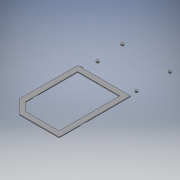
# Autodesk Inventor part: Backplate_V2
Saved by Autodesk Inventor 2016 SP2 (Build 200236200, 236)
## iProperties
Created: 2018-06-11
Part Number: Backplate_V2
Material: Generisch
Document SubType Name: Modeling
Designer: Nils
Density: 1 g/cm^3
Appearance: Vorgabe
Author: Nils
Autodesk Inventor part; units mm, degrees
ref_plane "YZ Plane" through (0, 0, 0) normal (1, 0, 0) x (0, 1, 0)
ref_plane "XZ Plane" through (0, 0, 0) normal (0, 1, 0) x (-1, 0, 0)
ref_plane "XY Plane" through (0, 0, 0) normal (0, 0, 1) x (1, 0, 0)
sketch "Skizze1" plane through (0, 0, 0) normal (0, 0, 1) x (1, 0, 0)
  line L0 (49.5001, 248.3761) -> (-49.5001, 248.3761) projected
  line L1 (49.5001, 95.1751) -> (49.5001, 248.3761) projected
  line L2 (-49.5001, 248.3761) -> (-49.5001, 95.1751) construction
  line L3 (-49.5001, 95.1751) -> (49.5001, 95.1751) construction
  line L4 (49.5001, 95.1751) -> (-20.5915, 95.1751)
  line L5 (-20.5915, 95.1751) -> (-49.5001, 124.0836)
  line L6 (-49.5001, 124.0836) -> (-49.5001, 248.3761)
  line L7 (-39.5001, 238.3761) -> (39.5001, 238.3761)
  line L8 (39.5001, 238.3761) -> (39.5001, 105.1751)
  line L9 (39.5001, 105.1751) -> (-19.2778, 105.1751)
  line L10 (-19.2778, 105.1751) -> (-39.5001, 125.3973)
  line L11 (-39.5001, 125.3973) -> (-39.5001, 238.3761)
  circle A0 centre (44.5001, 243.3761) radius 2.5 projected
  circle A1 centre (-44.5001, 243.3761) radius 2.5 projected
  circle A2 centre (-44.5001, 171.4345) radius 2.5 projected
  circle A3 centre (44.5001, 171.4345) radius 2.5 projected
  circle A4 centre (44.5001, 100.1751) radius 2.5 projected
  circle A5 centre (-20.9666, 110.5265) radius 1.75 projected
  circle A6 centre (-24.6237, 114.0565) radius 1.75 projected
  circle A7 centre (-44.8001, 100.0237) radius 1.75 projected
  circle A8 centre (-29.7001, 100.0237) radius 1.75 projected
  point P0 (0, 0)
  dimension "d0" = 135
  dimension "d1" = 8
  dimension "d3" = 10
  dimension "d4" = 10
  dimension "d5" = 10
  dimension "d6" = 10
  dimension "d22" = 2.5
  constraints: 16 end point, 3 perpendicular, 2 point on line, 1 collinear, 1 horizontal, 1 parallel
  measures "d0" angle of L5 L3
  measures "d1" distance between parallel lines of L5 L10
  measures "d3" distance between parallel lines of L3 L9
  measures "d4" distance between parallel lines of L1 L8
  measures "d5" distance between parallel lines of L2 L11
  measures "d6" distance between parallel lines of L0 L7
  measures "d22" distance from line of A6.centre L10
extrude "Extrusion1" add sketch "Skizze1" along normal blind 1.5 contours L1 L4 L5 L6 L0 | A0 | A1 | A2 | A3 | A4
sketch "Skizze2" plane through (0, 0, 0) normal (0, 0, -1) x (-1, 0, 0)
  circle A0 centre (-44.5001, 100.1751) radius 2.5 projected
  circle A1 centre (-44.5001, 171.4345) radius 2.5 projected
  circle A2 centre (-44.5001, 243.3761) radius 2.5 projected
  circle A3 centre (40.1569, 120.3973) radius 2.5 projected
  circle A4 centre (44.5001, 171.4345) radius 2.5 projected
  circle A5 centre (44.5001, 243.3761) radius 2.5 projected
  circle A6 centre (-44.5001, 100.1751) radius 2.4
  circle A7 centre (-44.5001, 171.4345) radius 2.4
  circle A8 centre (-44.5001, 243.3761) radius 2.4
  circle A9 centre (44.5001, 243.3761) radius 2.4
  circle A10 centre (44.5001, 171.4345) radius 2.4
  circle A11 centre (40.1569, 120.3973) radius 2.4
  dimension "d23" = 0.1
  dimension "d24" = 4.8
  dimension "d25" = 4.8
  dimension "d26" = 4.8
  dimension "d27" = 4.8
  dimension "d28" = 4.8
  dimension "d29" = 4.8
  constraints: 6 centre point, 5 coincident
  measures "d23" radial gap between concentric circles of A0 A6
  measures "d24" diameter of A6
  measures "d25" diameter of A7
  measures "d26" diameter of A8
  measures "d27" diameter of A9
  measures "d28" diameter of A10
  measures "d29" diameter of A11
extrude "Extrusion2" add sketch "Skizze2" along normal blind 2.6 contours A6 | A7 | A8 | A9 | A10 | A11
sketch "Skizze3" plane through (0, 0, 0) normal (0, 0, -1) x (-1, 0, 0)
  line L0 (-49.5001, 95.1751) -> (-49.5001, 248.3761) projected
  line L1 (-39.5001, 238.3761) -> (-39.5001, 105.1751) projected
  line L2 (-49.5001, 135.1751) -> (-39.5001, 135.1751)
  line L3 (-39.5001, 135.1751) -> (-39.5001, 145.1751)
  line L4 (-39.5001, 145.1751) -> (-49.5001, 145.1751)
  line L5 (-49.5001, 145.1751) -> (-49.5001, 135.1751)
  line L6 (39.5001, 238.3761) -> (39.5001, 125.3973) projected
  line L7 (49.5001, 248.3761) -> (49.5001, 124.0836) projected
  line L8 (39.5001, 135.1751) -> (49.5001, 135.1751)
  line L9 (49.5001, 135.1751) -> (49.5001, 145.1751)
  line L10 (49.5001, 145.1751) -> (39.5001, 145.1751)
  line L11 (39.5001, 145.1751) -> (39.5001, 135.1751)
  line L12 (39.5001, 125.3973) -> (19.2778, 105.1751) projected
  line L13 (20.692, 106.5893) -> (26.3489, 100.9324)
  line L14 (49.5001, 124.0836) -> (20.5915, 95.1751) projected
  line L15 (26.3489, 100.9324) -> (33.42, 108.0035)
  line L16 (33.42, 108.0035) -> (27.7631, 113.6604)
  line L17 (27.7631, 113.6604) -> (20.692, 106.5893)
  line L18 (20.5915, 95.1751) -> (-49.5001, 95.1751) projected
  point P0 (0, 0)
  dimension "d11" = 10
  dimension "d12" = 10
  dimension "d13" = 10
  dimension "d14" = 0
  dimension "d15" = 40
  dimension "d16" = 2
  constraints: 24 end point, 8 point on line, 4 parallel, 3 perpendicular, 2 horizontal, 1 collinear
  measures "d11" distance between parallel lines of L2 L4
  measures "d12" distance between parallel lines of L16 L13
  measures "d13" distance between parallel lines of L10 L8
  measures "d14" distance between parallel lines of L8 L2
  measures "d15" distance between parallel lines of L18 L2
  measures "d16" distance from line of L12.end L13
extrude "Extrusion3" cut sketch "Skizze3" against normal blind 1 contours L0 L4 L1 L2 | L13 L12 L16 L14 | L8 L6 L10 L7
equation "\"d4\" = d3"
equation "\"d5\" = d3"
equation "\"d6\" = d3"
equation "\"d25\" = d24"
equation "\"d26\" = d24"
equation "\"d27\" = d24"
equation "\"d28\" = d24"
equation "\"d29\" = d24"
equation "\"d12\" = d11"
equation "\"d13\" = d11"
